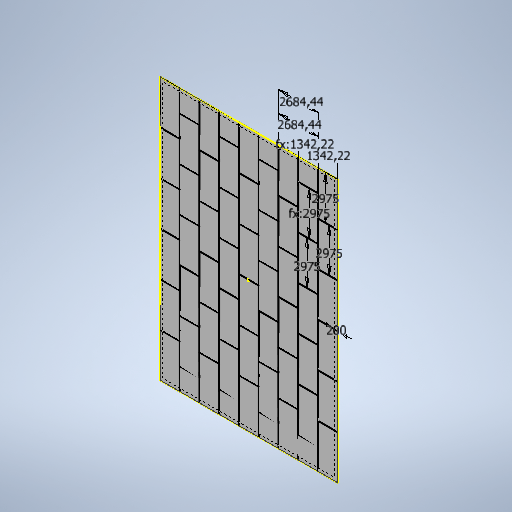
# Autodesk Inventor part: GBK bottom
Saved by Autodesk Inventor 2026 (Build 300175000, 175)
## iProperties
Created: 2026-04-17
Part Number: GBK bottom
Material: Generic
Document SubType Name: Sheet Metal
Designer: admin
Density: 1 g/cm^3
Sheet Metal Rule: По умолчанию_мм
Appearance: Default
Author: admin
Autodesk Inventor part; units mm, degrees
ref_plane "YZ Plane" through (0, 0, 0) normal (1, 0, 0) x (0, 1, 0)
ref_plane "XZ Plane" through (0, 0, 0) normal (0, 1, 0) x (-1, 0, 0)
ref_plane "XY Plane" through (0, 0, 0) normal (0, 0, 1) x (1, 0, 0)
sketch "Sketch1" plane through (0, 0, 0) normal (0, 0, 1) x (1, 0, 0)
  line L0 (6040, -8925) -> (-6040, -8925)
  line L1 (-6040, -8925) -> (-6040, 8925)
  line L2 (-6040, 8925) -> (6040, 8925)
  line L3 (6040, 8925) -> (6040, -8925)
  line L4 (6040, -8925) -> (-6040, 8925) construction
  line L5 (-6040, -8925) -> (6040, 8925) construction
  point P0 (0, 0)
  dimension "d0" = 12080
  dimension "d1" = 17850
  measures "d0" distance of L1.end L2.end
  measures "d1" distance of L0.end L1.end
extrude "Plate1" add sketch "Sketch1" along normal blind 6
sketch "Эскиз7" plane through (0, 0, 6) normal (0, 0, 1) x (1, 0, 0)
  line L0 (6040, 8925) -> (6040, -8925) projected
  line L1 (-6040, 8925) -> (6040, 8925) projected
  line L2 (-6040, -8925) -> (-6040, 8925) projected
  line L3 (6040, -8925) -> (-6040, -8925) projected
  line L4 (6040, 8925) -> (4697.78, 8925)
  line L5 (4697.78, 8925) -> (4697.78, 5950)
  line L6 (4697.78, 5950) -> (6040, 5950)
  line L7 (6040, 5950) -> (6040, 8925)
  line L8 (4697.78, 2975) -> (6040, 2975)
  line L9 (4697.78, 5950) -> (4697.78, 2975)
  line L10 (6040, 5950) -> (4697.78, 5950)
  line L11 (6040, 2975) -> (6040, 5950)
  line L12 (4697.78, 0) -> (6040, 0)
  line L13 (4697.78, 2975) -> (4697.78, 0)
  line L14 (6040, 2975) -> (4697.78, 2975)
  line L15 (6040, 0) -> (6040, 2975)
  line L16 (4697.78, -2975) -> (6040, -2975)
  line L17 (4697.78, 0) -> (4697.78, -2975)
  line L18 (6040, 0) -> (4697.78, 0)
  line L19 (6040, -2975) -> (6040, 0)
  line L20 (4697.78, -5950) -> (6040, -5950)
  line L21 (4697.78, -2975) -> (4697.78, -5950)
  line L22 (6040, -2975) -> (4697.78, -2975)
  line L23 (6040, -5950) -> (6040, -2975)
  line L24 (4697.78, -8925) -> (6040, -8925)
  line L25 (4697.78, -5950) -> (4697.78, -8925)
  line L26 (6040, -5950) -> (4697.78, -5950)
  line L27 (6040, -8925) -> (6040, -5950)
  line L28 (4697.78, 7437.5) -> (3355.56, 7437.5)
  line L29 (3355.56, 7437.5) -> (3355.56, 4462.5)
  line L30 (3355.56, 4462.5) -> (4697.78, 4462.5)
  line L31 (4697.78, 4462.5) -> (4697.78, 7437.5)
  line L32 (3355.56, 1487.5) -> (4697.78, 1487.5)
  line L33 (4697.78, 1487.5) -> (4697.78, 4462.5)
  line L34 (4697.78, 4462.5) -> (3355.56, 4462.5)
  line L35 (3355.56, 4462.5) -> (3355.56, 1487.5)
  line L36 (3355.56, -1487.5) -> (4697.78, -1487.5)
  line L37 (4697.78, -1487.5) -> (4697.78, 1487.5)
  line L38 (4697.78, 1487.5) -> (3355.56, 1487.5)
  line L39 (3355.56, 1487.5) -> (3355.56, -1487.5)
  line L40 (3355.56, -4462.5) -> (4697.78, -4462.5)
  line L41 (4697.78, -4462.5) -> (4697.78, -1487.5)
  line L42 (4697.78, -1487.5) -> (3355.56, -1487.5)
  line L43 (3355.56, -1487.5) -> (3355.56, -4462.5)
  line L44 (3355.56, -7437.5) -> (4697.78, -7437.5)
  line L45 (4697.78, -7437.5) -> (4697.78, -4462.5)
  line L46 (4697.78, -4462.5) -> (3355.56, -4462.5)
  line L47 (3355.56, -4462.5) -> (3355.56, -7437.5)
  line L48 (2013.34, 2975) -> (3355.56, 2975)
  line L49 (2013.34, 1487.5) -> (2013.34, 4462.5)
  line L50 (3355.56, 0) -> (3355.56, 2975)
  line L51 (2013.34, 2975) -> (2013.34, 0)
  line L52 (2013.34, -1487.5) -> (2013.34, 1487.5)
  line L53 (2013.34, 0) -> (3355.56, 0)
  line L54 (2013.34, -2975) -> (3355.56, -2975)
  line L55 (2013.34, 0) -> (2013.34, -2975)
  line L56 (3355.56, 0) -> (2013.34, 0)
  line L57 (3355.56, -2975) -> (3355.56, 0)
  line L58 (2013.34, -5950) -> (3355.56, -5950)
  line L59 (2013.34, -2975) -> (2013.34, -5950)
  line L60 (3355.56, -5950) -> (3355.56, -2975)
  line L61 (3355.56, -2975) -> (2013.34, -2975)
  line L62 (2013.34, -4462.5) -> (2013.34, -1487.5)
  line L63 (3355.56, -5950) -> (2013.34, -5950)
  line L64 (2013.34, -7437.5) -> (2013.34, -4462.5)
  line L65 (2013.34, -5950) -> (2013.34, -8925)
  line L66 (3355.56, -8925) -> (3355.56, -5950)
  line L67 (2013.34, -8925) -> (3355.56, -8925)
  line L68 (3355.56, 8925) -> (2013.34, 8925)
  line L69 (2013.34, 8925) -> (2013.34, 5950)
  line L70 (2013.34, 5950) -> (3355.56, 5950)
  line L71 (3355.56, 5950) -> (3355.56, 8925)
  line L72 (3355.56, 2975) -> (2013.34, 2975)
  line L73 (2013.34, 5950) -> (2013.34, 2975)
  line L74 (3355.56, 5950) -> (2013.34, 5950)
  line L75 (3355.56, 2975) -> (3355.56, 5950)
  line L76 (2013.34, 4462.5) -> (2013.34, 7437.5)
  line L77 (-671.1, 2975) -> (671.12, 2975)
  line L78 (-671.1, 1487.5) -> (-671.1, 4462.5)
  line L79 (671.12, 0) -> (671.12, 2975)
  line L80 (-671.1, 2975) -> (-671.1, 0)
  line L81 (-671.1, -1487.5) -> (-671.1, 1487.5)
  line L82 (-671.1, 0) -> (671.12, 0)
  line L83 (-671.1, -2975) -> (671.12, -2975)
  line L84 (-671.1, 0) -> (-671.1, -2975)
  line L85 (671.12, 0) -> (-671.1, 0)
  line L86 (671.12, -2975) -> (671.12, 0)
  line L87 (-671.1, -5950) -> (671.12, -5950)
  line L88 (-671.1, -2975) -> (-671.1, -5950)
  line L89 (671.12, -5950) -> (671.12, -2975)
  line L90 (671.12, -2975) -> (-671.1, -2975)
  line L91 (-671.1, -4462.5) -> (-671.1, -1487.5)
  line L92 (671.12, -5950) -> (-671.1, -5950)
  line L93 (-671.1, -7437.5) -> (-671.1, -4462.5)
  line L94 (-671.1, -5950) -> (-671.1, -8925)
  line L95 (671.12, -8925) -> (671.12, -5950)
  line L96 (-671.1, -8925) -> (671.12, -8925)
  line L97 (671.12, 8925) -> (-671.1, 8925)
  line L98 (-671.1, 8925) -> (-671.1, 5950)
  line L99 (-671.1, 5950) -> (671.12, 5950)
  line L100 (671.12, 5950) -> (671.12, 8925)
  line L101 (671.12, 2975) -> (-671.1, 2975)
  line L102 (-671.1, 5950) -> (-671.1, 2975)
  line L103 (671.12, 5950) -> (-671.1, 5950)
  line L104 (671.12, 2975) -> (671.12, 5950)
  line L105 (-671.1, 4462.5) -> (-671.1, 7437.5)
  line L106 (-3355.54, 2975) -> (-2013.32, 2975)
  line L107 (-3355.54, 1487.5) -> (-3355.54, 4462.5)
  line L108 (-2013.32, 0) -> (-2013.32, 2975)
  line L109 (-3355.54, 2975) -> (-3355.54, 0)
  line L110 (-3355.54, -1487.5) -> (-3355.54, 1487.5)
  line L111 (-3355.54, 0) -> (-2013.32, 0)
  line L112 (-3355.54, -2975) -> (-2013.32, -2975)
  line L113 (-3355.54, 0) -> (-3355.54, -2975)
  line L114 (-2013.32, 0) -> (-3355.54, 0)
  line L115 (-2013.32, -2975) -> (-2013.32, 0)
  line L116 (-3355.54, -5950) -> (-2013.32, -5950)
  line L117 (-3355.54, -2975) -> (-3355.54, -5950)
  line L118 (-2013.32, -5950) -> (-2013.32, -2975)
  line L119 (-2013.32, -2975) -> (-3355.54, -2975)
  line L120 (-3355.54, -4462.5) -> (-3355.54, -1487.5)
  line L121 (-2013.32, -5950) -> (-3355.54, -5950)
  line L122 (-3355.54, -7437.5) -> (-3355.54, -4462.5)
  line L123 (-3355.54, -5950) -> (-3355.54, -8925)
  line L124 (-2013.32, -8925) -> (-2013.32, -5950)
  line L125 (-3355.54, -8925) -> (-2013.32, -8925)
  line L126 (-2013.32, 8925) -> (-3355.54, 8925)
  line L127 (-3355.54, 8925) -> (-3355.54, 5950)
  line L128 (-3355.54, 5950) -> (-2013.32, 5950)
  line L129 (-2013.32, 5950) -> (-2013.32, 8925)
  line L130 (-2013.32, 2975) -> (-3355.54, 2975)
  line L131 (-3355.54, 5950) -> (-3355.54, 2975)
  line L132 (-2013.32, 5950) -> (-3355.54, 5950)
  line L133 (-2013.32, 2975) -> (-2013.32, 5950)
  line L134 (-3355.54, 4462.5) -> (-3355.54, 7437.5)
  line L135 (-6039.98, 2975) -> (-4697.76, 2975)
  line L136 (-6039.98, 1487.5) -> (-6039.98, 4462.5)
  line L137 (-4697.76, 0) -> (-4697.76, 2975)
  line L138 (-6039.98, 2975) -> (-6039.98, 0)
  line L139 (-6039.98, -1487.5) -> (-6039.98, 1487.5)
  line L140 (-6039.98, 0) -> (-4697.76, 0)
  line L141 (-6039.98, -2975) -> (-4697.76, -2975)
  line L142 (-6039.98, 0) -> (-6039.98, -2975)
  line L143 (-4697.76, 0) -> (-6039.98, 0)
  line L144 (-4697.76, -2975) -> (-4697.76, 0)
  line L145 (-6039.98, -5950) -> (-4697.76, -5950)
  line L146 (-6039.98, -2975) -> (-6039.98, -5950)
  line L147 (-4697.76, -5950) -> (-4697.76, -2975)
  line L148 (-4697.76, -2975) -> (-6039.98, -2975)
  line L149 (-6039.98, -4462.5) -> (-6039.98, -1487.5)
  line L150 (-4697.76, -5950) -> (-6039.98, -5950)
  line L151 (-6039.98, -7437.5) -> (-6039.98, -4462.5)
  line L152 (-6039.98, -5950) -> (-6039.98, -8925)
  line L153 (-4697.76, -8925) -> (-4697.76, -5950)
  line L154 (-6039.98, -8925) -> (-4697.76, -8925)
  line L155 (-4697.76, 8925) -> (-6039.98, 8925)
  line L156 (-6039.98, 8925) -> (-6039.98, 5950)
  line L157 (-6039.98, 5950) -> (-4697.76, 5950)
  line L158 (-4697.76, 5950) -> (-4697.76, 8925)
  line L159 (-4697.76, 2975) -> (-6039.98, 2975)
  line L160 (-6039.98, 5950) -> (-6039.98, 2975)
  line L161 (-4697.76, 5950) -> (-6039.98, 5950)
  line L162 (-4697.76, 2975) -> (-4697.76, 5950)
  line L163 (-6039.98, 4462.5) -> (-6039.98, 7437.5)
  line L164 (2013.34, 2975) -> (2013.34, 0)
  line L165 (671.12, 1487.5) -> (2013.34, 1487.5)
  line L166 (2013.34, 1487.5) -> (671.12, 1487.5)
  line L167 (671.12, 0) -> (671.12, 2975)
  line L168 (2013.34, -2975) -> (2013.34, -5950)
  line L169 (671.12, -5950) -> (671.12, -2975)
  line L170 (671.12, -4462.5) -> (671.12, -7437.5)
  line L171 (671.12, -7437.5) -> (2013.34, -7437.5)
  line L172 (2013.34, -7437.5) -> (2013.34, -4462.5)
  line L173 (2013.34, 5950) -> (2013.34, 2975)
  line L174 (2013.34, 4462.5) -> (671.12, 4462.5)
  line L175 (671.12, 2975) -> (671.12, 5950)
  line L176 (671.12, 4462.5) -> (671.12, 1487.5)
  line L177 (2013.34, 1487.5) -> (2013.34, 4462.5)
  line L178 (671.12, 4462.5) -> (2013.34, 4462.5)
  line L179 (671.12, -1487.5) -> (2013.34, -1487.5)
  line L180 (671.12, -4462.5) -> (2013.34, -4462.5)
  line L181 (2013.34, -4462.5) -> (2013.34, -1487.5)
  line L182 (2013.34, -1487.5) -> (671.12, -1487.5)
  line L183 (671.12, -1487.5) -> (671.12, -4462.5)
  line L184 (2013.34, -4462.5) -> (671.12, -4462.5)
  line L185 (2013.34, -1487.5) -> (2013.34, 1487.5)
  line L186 (671.12, 1487.5) -> (671.12, -1487.5)
  line L187 (2013.34, 0) -> (2013.34, -2975)
  line L188 (671.12, -2975) -> (671.12, 0)
  line L189 (2013.34, 8925) -> (2013.34, 5950)
  line L190 (671.12, 7437.5) -> (671.12, 4462.5)
  line L191 (2013.34, 4462.5) -> (2013.34, 7437.5)
  line L192 (2013.34, 7437.5) -> (671.12, 7437.5)
  line L193 (671.12, 5950) -> (671.12, 8925)
  line L194 (2013.34, -5950) -> (2013.34, -8925)
  line L195 (671.12, -8925) -> (671.12, -5950)
  line L196 (-671.1, 2975) -> (-671.1, 0)
  line L197 (-2013.32, 1487.5) -> (-671.1, 1487.5)
  line L198 (-671.1, 1487.5) -> (-2013.32, 1487.5)
  line L199 (-2013.32, 0) -> (-2013.32, 2975)
  line L200 (-671.1, -2975) -> (-671.1, -5950)
  line L201 (-2013.32, -5950) -> (-2013.32, -2975)
  line L202 (-2013.32, -4462.5) -> (-2013.32, -7437.5)
  line L203 (-2013.32, -7437.5) -> (-671.1, -7437.5)
  line L204 (-671.1, -7437.5) -> (-671.1, -4462.5)
  line L205 (-671.1, 5950) -> (-671.1, 2975)
  line L206 (-671.1, 4462.5) -> (-2013.32, 4462.5)
  line L207 (-2013.32, 2975) -> (-2013.32, 5950)
  line L208 (-2013.32, 4462.5) -> (-2013.32, 1487.5)
  line L209 (-671.1, 1487.5) -> (-671.1, 4462.5)
  line L210 (-2013.32, 4462.5) -> (-671.1, 4462.5)
  line L211 (-2013.32, -1487.5) -> (-671.1, -1487.5)
  line L212 (-2013.32, -4462.5) -> (-671.1, -4462.5)
  line L213 (-671.1, -4462.5) -> (-671.1, -1487.5)
  line L214 (-671.1, -1487.5) -> (-2013.32, -1487.5)
  line L215 (-2013.32, -1487.5) -> (-2013.32, -4462.5)
  line L216 (-671.1, -4462.5) -> (-2013.32, -4462.5)
  line L217 (-671.1, -1487.5) -> (-671.1, 1487.5)
  line L218 (-2013.32, 1487.5) -> (-2013.32, -1487.5)
  line L219 (-671.1, 0) -> (-671.1, -2975)
  line L220 (-2013.32, -2975) -> (-2013.32, 0)
  line L221 (-671.1, 8925) -> (-671.1, 5950)
  line L222 (-2013.32, 7437.5) -> (-2013.32, 4462.5)
  line L223 (-671.1, 4462.5) -> (-671.1, 7437.5)
  line L224 (-671.1, 7437.5) -> (-2013.32, 7437.5)
  line L225 (-2013.32, 5950) -> (-2013.32, 8925)
  line L226 (-671.1, -5950) -> (-671.1, -8925)
  line L227 (-2013.32, -8925) -> (-2013.32, -5950)
  line L228 (-3355.54, 2975) -> (-3355.54, 0)
  line L229 (-4697.76, 1487.5) -> (-3355.54, 1487.5)
  line L230 (-3355.54, 1487.5) -> (-4697.76, 1487.5)
  line L231 (-4697.76, 0) -> (-4697.76, 2975)
  line L232 (-3355.54, -2975) -> (-3355.54, -5950)
  line L233 (-4697.76, -5950) -> (-4697.76, -2975)
  line L234 (-4697.76, -4462.5) -> (-4697.76, -7437.5)
  line L235 (-4697.76, -7437.5) -> (-3355.54, -7437.5)
  line L236 (-3355.54, -7437.5) -> (-3355.54, -4462.5)
  line L237 (-3355.54, 5950) -> (-3355.54, 2975)
  line L238 (-3355.54, 4462.5) -> (-4697.76, 4462.5)
  line L239 (-4697.76, 2975) -> (-4697.76, 5950)
  line L240 (-4697.76, 4462.5) -> (-4697.76, 1487.5)
  line L241 (-3355.54, 1487.5) -> (-3355.54, 4462.5)
  line L242 (-4697.76, 4462.5) -> (-3355.54, 4462.5)
  line L243 (-4697.76, -1487.5) -> (-3355.54, -1487.5)
  line L244 (-4697.76, -4462.5) -> (-3355.54, -4462.5)
  line L245 (-3355.54, -4462.5) -> (-3355.54, -1487.5)
  line L246 (-3355.54, -1487.5) -> (-4697.76, -1487.5)
  line L247 (-4697.76, -1487.5) -> (-4697.76, -4462.5)
  line L248 (-3355.54, -4462.5) -> (-4697.76, -4462.5)
  line L249 (-3355.54, -1487.5) -> (-3355.54, 1487.5)
  line L250 (-4697.76, 1487.5) -> (-4697.76, -1487.5)
  line L251 (-3355.54, 0) -> (-3355.54, -2975)
  line L252 (-4697.76, -2975) -> (-4697.76, 0)
  line L253 (-3355.54, 8925) -> (-3355.54, 5950)
  line L254 (-4697.76, 7437.5) -> (-4697.76, 4462.5)
  line L255 (-3355.54, 4462.5) -> (-3355.54, 7437.5)
  line L256 (-3355.54, 7437.5) -> (-4697.76, 7437.5)
  line L257 (-4697.76, 5950) -> (-4697.76, 8925)
  line L258 (-3355.54, -5950) -> (-3355.54, -8925)
  line L259 (-4697.76, -8925) -> (-4697.76, -5950)
  line L260 (5840, -8725) -> (5840, 8725) construction
  line L261 (5840, 8725) -> (-5840, 8725) construction
  line L262 (-5840, 8725) -> (-5840, -8725) construction
  line L263 (-5840, -8725) -> (5840, -8725) construction
  point P0 (0, 0)
  dimension "d104" = 2975
  dimension "d105" = 1342.22
  dimension "d108" = 2975
  dimension "d113" = 1342.22
  dimension "d114" = 2975
  dimension "d117" = 2975
  dimension "d124" = 2684.44
  dimension "d131" = 2684.44
  dimension "d136" = 200
  constraints: 520 end point, 4 horizontal, 4 parallel, 2 perpendicular, 2 vertical, 1 midpoint, 555 other
  measures "d104" distance between parallel lines of L6 L1
  measures "d105" distance between parallel lines of L0 L5
  measures "d108" distance of L5.end L8.start
  measures "d113" distance between parallel lines of L29 L5
  measures "d114" distance between parallel lines of L28 L30
  measures "d117" distance of L29.end L32.start
  measures "d124" distance of L8.start L48.start
  measures "d131" distance of L8.start L173.end
  measures "d136" distance between parallel lines of L0 L260
equation "\"d113\" = d105"
equation "\"d114\" = d104"
equation "\"d2\" = Thickness"
equation "\"BendRadius\" = Thickness"
equation "\"BendReliefWidth\" = Thickness"
equation "\"BendReliefDepth\" = 0.5 * Thickness"
equation "\"CornerReliefSize\" = 4 * Thickness"
equation "\"MinimumRemnant\" = 2 * Thickness"
equation "\"TransitionRadius\" = BendRadius"
equation "\"JacobiRadiusSize\" = BendRadius"
equation "\"GapSize\" = Thickness"
equation "\"Thickness\" = 6"
body "Solid1"
